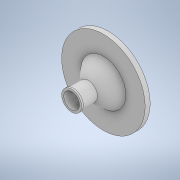
# Autodesk Inventor part: Крышка_быстроходного
Saved by Autodesk Inventor 2021 (Build 250183000, 183)
## iProperties
Created: 2023-03-23
Part Number: Крышка_быстроходного
Material: Типовые
Document SubType Name: Modeling
Designer: gdevc
Density: 1 g/cm^3
Appearance: По умолчанию
Author: gdevc
Autodesk Inventor part; units mm, degrees
ref_plane "YZ Plane" through (0, 0, 0) normal (1, 0, 0) x (0, 1, 0)
ref_plane "XZ Plane" through (0, 0, 0) normal (0, 1, 0) x (-1, 0, 0)
ref_plane "XY Plane" through (0, 0, 0) normal (0, 0, 1) x (1, 0, 0)
sketch "Эскиз1" plane through (0, 0, 0) normal (1, 0, 0) x (0, 1, 0)
  line L0 (0, 0) -> (0, -73.7994) construction
  line L1 (23.5, 0) -> (23.5, -56.0436)
  line L2 (23.5, -56.0436) -> (68.5622, -107)
  line L3 (125, -110.9688) -> (125, -95)
  line L4 (125, -95) -> (67.2948, -95)
  line L5 (67.2948, -95) -> (27.5, -50)
  line L6 (27.5, -50) -> (27.5, -5)
  line L7 (27.5, -5) -> (30, -5)
  line L8 (30, -5) -> (30, 0)
  line L9 (30, 0) -> (23.5, 0)
  line L10 (68.5622, -107) -> (90, -107)
  line L11 (90, -107) -> (90, -110)
  line L12 (90, -110) -> (125, -110)
  line L13 (125, -110) -> (125, -110.9688)
  dimension "d13" = 47
  dimension "d14" = 180
  dimension "d15" = 250
  dimension "d16" = 7
  dimension "d18" = 0
  dimension "d19" = 15
  dimension "d20" = 3
  dimension "d21" = 60
  dimension "d22" = 4
  dimension "d23" = 5
  dimension "d24" = 50
  dimension "d25" = 60
  constraints: 28 end point, 7 perpendicular, 2 parallel, 2 vertical, 1 horizontal
  measures "d13" diameter of L1 L0
  measures "d14" diameter of L11 L0
  measures "d15" diameter of L13 L0
  measures "d16" distance between parallel lines of L2 L5
  measures "d18" distance from line of L0.start L9
  measures "d19" distance between parallel lines of L12 L4
  measures "d20" distance of L10.end L11.end
  measures "d21" diameter of L8 L0
  measures "d22" distance between parallel lines of L1 L6
  measures "d23" distance between parallel lines of L9 L7
  measures "d24" vertical distance of L0.start L5.end
  measures "d25" distance from line of L12 L5.end
revolve "Вращение1" add sketch "Эскиз1" angle 360 about axis through (0, 0, 0) along (0, 0, -1)
